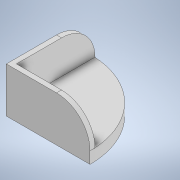
# Autodesk Inventor part: euro_box_corner_r
Saved by Autodesk Inventor 2020 (Build 240168000, 168)
## iProperties
Created: 2019-11-21
Part Number: euro_box_corner_r
Material: Generic
Document SubType Name: Modeling
Designer: NILY
Density: 1 g/cm^3
Appearance: Default
Author: NILY
Autodesk Inventor part; units mm, degrees
ref_plane "YZ Plane" through (0, 0, 0) normal (1, 0, 0) x (0, 1, 0)
ref_plane "XZ Plane" through (0, 0, 0) normal (0, 1, 0) x (-1, 0, 0)
ref_plane "XY Plane" through (0, 0, 0) normal (0, 0, 1) x (1, 0, 0)
sketch "Sketch1" plane through (0, 0, 0) normal (0, 1, 0) x (-1, 0, 0)
  circle A0 centre (0, 0) radius 50
  dimension "d0" = 100
  constraints: 1 centre point, 1 coincident
  measures "d0" diameter of A0
extrude "Extrusion1" add sketch "Sketch1" along normal blind 7
sketch "Sketch2" plane through (0, 7, 0) normal (0, 1, 0) x (1, 0, 0)
  line L0 (0, 0) -> (50, 0)
  line L1 (50, 0) -> (50, 3)
  line L2 (50, 3) -> (0, 3)
  line L3 (0, 3) -> (0, 0)
  dimension "d3" = 50
  dimension "d4" = 3
  constraints: 8 end point, 2 parallel, 1 horizontal, 1 perpendicular
  measures "d3" distance of L2.end L1.end
  measures "d4" distance of L1.end L0.end
extrude "Extrusion2" add sketch "Sketch2" along normal blind 20
sketch "Sketch3" plane through (0, 7, 0) normal (0, 1, 0) x (1, 0, 0)
  line L0 (0, 3) -> (0, 0) projected
  line L1 (0, 0) -> (3, 0)
  line L2 (3, 0) -> (3, 50)
  line L3 (3, 50) -> (0, 50)
  line L4 (0, 50) -> (0, 0)
  dimension "d7" = 3
  dimension "d8" = 50
  constraints: 8 end point, 2 parallel, 1 horizontal, 1 perpendicular
  measures "d7" distance of L3.end L2.end
  measures "d8" distance of L2.end L1.end
extrude "Extrusion3" add sketch "Sketch3" along normal blind 20
sketch "Sketch4" plane through (0, 7, 0) normal (0, 1, 0) x (1, 0, 0)
  line L0 (0, 0) -> (0, 50) projected
  line L1 (0, 50) -> (-50, 50)
  line L2 (-50, 50) -> (-50, -50)
  line L3 (-50, -50) -> (0, -50)
  line L4 (0, -50) -> (0, 50)
  line L5 (50, 0) -> (0, 0) projected
  line L6 (0, 0) -> (50, 0)
  line L7 (50, 0) -> (50, -50)
  line L8 (50, -50) -> (0, -50)
  line L9 (0, -50) -> (0, 0)
  dimension "d11" = 50
  dimension "d12" = 100
  dimension "d13" = 50
  dimension "d14" = 50
  constraints: 16 end point, 4 parallel, 2 horizontal, 2 perpendicular
  measures "d11" distance of L3.end L2.end
  measures "d12" distance of L2.end L1.end
  measures "d13" distance of L7.end L8.end
  measures "d14" distance of L6.end L7.end
extrude "Extrusion4" cut sketch "Sketch4" against normal blind 7
sketch "Sketch5" plane through (0, 7, 0) normal (0, 1, 0) x (1, 0, 0)
  line L0 (3, 49.9099) -> (3, 3) projected
  line L1 (3, 3) -> (49.9099, 3) projected
  point P0 (0, 0)
  point P1 (23, 13)
  dimension "d24" = 20
  dimension "d25" = 10
  measures "d24" distance from line of point (23, 13) L0
  measures "d25" distance from line of point (23, 13) L1
hole "Hole1" at (23, 7, -13) direction (0, -1, 0) diameter 6.5 end through all counterbore diameter 10.5 counterbore depth 5
fillet "Fillet1" radius 20 1 edges at (1.5, 27, -50)
fillet "Fillet2" radius 20 1 edges at (50, 27, -1.5)
body "Solid1"
